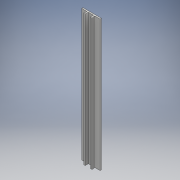
# Autodesk Inventor part: Estrutura - suporteCalha
Saved by Autodesk Inventor 2017 (Build 210142000, 142)
## iProperties
Created: 2020-10-25
Part Number: Estrutura - suporteCalha
Material: Generic
Document SubType Name: Modeling
Designer: ale
Density: 1 g/cm^3
Appearance: Default
Author: ale
Autodesk Inventor part; units mm, degrees
ref_plane "YZ Plane" through (0, 0, 0) normal (1, 0, 0) x (0, 1, 0)
ref_plane "XZ Plane" through (0, 0, 0) normal (0, 1, 0) x (-1, 0, 0)
ref_plane "XY Plane" through (0, 0, 0) normal (0, 0, 1) x (1, 0, 0)
sketch "Sketch1" plane through (0, 0, 0) normal (0, 0, 1) x (1, 0, 0)
  line L0 (-7, 2.5) -> (7, 2.5)
  line L1 (-3, 1.5) -> (-3, 0)
  line L2 (-3.3, 0) -> (-3, 0)
  line L3 (-3, 1.5) -> (-7, 1.5)
  line L4 (-7, 1.5) -> (-7, 2.5)
  line L5 (0, -2.5) -> (0, 2.5)
  line L6 (-3.3, 0) -> (-3.3, -0.6)
  line L7 (-2, 1.5) -> (-2, -0.9)
  line L8 (-3, -0.9) -> (-2, -0.9)
  line L9 (3, 1.5) -> (3, 0)
  line L10 (3, 1.5) -> (7, 1.5)
  line L11 (3.3, 0) -> (3.3, -0.6)
  line L12 (2, 1.5) -> (2, -0.9)
  line L13 (3, -0.9) -> (2, -0.9)
  line L14 (-2, 1.5) -> (2, 1.5)
  line L15 (3.3, 0) -> (3, 0)
  line L16 (7, 1.5) -> (7, 2.5)
  line L17 (-3, 0) -> (3, 0)
  line L18 (-3.3, -0.6) -> (-3, -0.9)
  line L19 (3.3, -0.6) -> (3, -0.9)
  point P0 (0, 0)
  point P1 (0, 0)
  point P2 (0, 0)
  dimension "d10" = 1
  dimension "d12" = 2
  dimension "d13" = 0.9
  dimension "d15" = 3.3
  dimension "d17" = 3.3
  dimension "d18" = 7
  dimension "d19" = 1.5
  dimension "d20" = 1.5
  dimension "d22" = 2.5
  constraints: 40 end point, 8 symmetric about line, 4 horizontal, 3 midpoint, 2 coincident, 2 perpendicular, 1 parallel, 1 vertical
  measures "d10" distance between parallel lines of L1 L7
  measures "d12" distance between parallel lines of L12 L5
  measures "d13" distance between parallel lines of L8 L17
  measures "d15" distance between parallel lines of L6 L5
  measures "d17" distance of point (0, 0) L2.start
  measures "d18" distance from line of point (0, 0) L4
  measures "d19" distance from line of point (0, 0) L10
  measures "d20" distance from line of point (0, 0) L14
  measures "d22" vertical distance of point (0, 0) L0.end
extrude "Extrusion1" add sketch "Sketch1" along normal blind 100 contours L0 L5 L14 L7 L17 L1 L3 L4 | L0 L16 L10 L9 L17 L12 L14 L5 | L17 L7 L8 L18 L6 L2 | L17 L15 L11 L19 L13 L12
body "Solid1"
